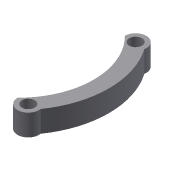
# Autodesk Inventor part: bar_mid
Saved by Autodesk Inventor 2018 (Build 220112000, 112)
## iProperties
Created: 2018-08-17
Part Number: bar_mid
Material: Generic
Document SubType Name: Modeling
Designer: Bardo91
Density: 1 g/cm^3
Appearance: Default
Author: Bardo91
Autodesk Inventor part; units mm, degrees
note: some values were not read from the file. Chosen so that the rebuilt part matches the saved one: sketch regions of "Extrusion1".
ref_plane "YZ Plane" through (0, 0, 0) normal (1, 0, 0) x (0, 1, 0)
ref_plane "XZ Plane" through (0, 0, 0) normal (0, 1, 0) x (-1, 0, 0)
ref_plane "XY Plane" through (0, 0, 0) normal (0, 0, 1) x (1, 0, 0)
sketch "Sketch1" plane through (0, 0, 0) normal (0, 0, 1) x (1, 0, 0)
  circle A0 centre (0, 0) radius 1.5
  circle A1 centre (0, 25) radius 1.5
  arc A2 (2.4636, 24.5748) -> (0, 22.5) centre (0, 25) ccw
  arc A3 (-2.5, 0) -> (-0.4252, 2.4636) centre (0, 0) ccw
  line L0 (0, 16.5) -> (0, 25)
  arc A4 (0, -2.5) -> (0, 27.5) centre (-14.8423, 12.5) ccw
  arc A5 (-2.5, 0) -> (-2.5, 25) centre (-14.8423, 12.5) ccw
  dimension "d0" = 3
  dimension "d3" = 25
  dimension "d4" = 3
  dimension "d5" = 5
  dimension "d6" = 5
  constraints: 13 point on circle, 6 centre point, 4 coincident, 2 end point, 1 concentric, 1 point on line, 1 vertical
  measures "d0" diameter of A0
  measures "d3" distance of A0.centre L0.end
  measures "d4" diameter of A1
  measures "d5" diameter of A2
  measures "d6" diameter of A3
extrude "Extrusion1" add sketch "Sketch1" along normal blind 5 contours A4 A2 | A4 A3 A5 L0 A2 | A4 A3 A5 | A3 A4 | A2 L0 A5
body "Solid1"
